HapticCoverMold (Autodesk Fusion 360 design; units mm, degrees)
Autodesk Fusion 360 part; units mm, degrees
sketch "Sketch1" plane through (0, 0, 0) normal (0, 0, 1) x (1, 0, 0) in component "Haptic Motor"
  circle A0 centre (0, 0) radius 5.2
  dimension "d1" = 10.4
  constraint coincident A0.centre origin
  measures "d1" diameter of A0
extrude "Extrude1" add sketch "Sketch1" along normal blind 6 makes body 1 in component "Haptic Motor"
sketch "Sketch1 (2)" plane through (0, 0, 0) normal (0, 0, 1) x (1, 0, 0) in component "Haptic Cover"
  circle A0 centre (0, 0) radius 5.2
  circle A1 centre (0, 0) radius 6.7
  dimension "d4" = 1.5
extrude "Extrude1'" add sketch "Sketch1 (2)" along normal blind 6 separate body makes body 2 in component "Haptic Cover"
extrude "Extrude2" add sketch "Sketch1 (2)" against normal blind 1.5 contours A0 | A1 bodies 2 in component "Haptic Cover"
sketch "Sketch1 (3)" plane through (0, 0, 0) normal (0, 1, 0) x (1, 0, 0) in component "Mold"
  line L0 (9.593, -10.0264) -> (-9.2463, -10.0264)
  line L1 (-9.2463, -10.0264) -> (-9.2463, 7.0138)
  line L2 (-9.2463, 7.0138) -> (9.593, 7.0138)
  line L3 (9.593, 7.0138) -> (9.593, -10.0264)
  constraint horizontal L0
  constraint vertical L1
  constraint horizontal L2
  constraint vertical L3
extrude "Extrude1''" add sketch "Sketch1 (3)" along normal mid plane 22 separate body makes body 3 in component "Mold"
ref_plane "WorkPlane1" through (0, 0, -1.5) normal (0, 0, -1) x (-1, 0, 0) in component "Mold"
combine "Combine1" operation cut target body 3 tool bodies 2 keep tools in component "Mold"
split "Split1" by plane through (0, 0, -1.5) normal (0, 0, -1) bodies 3 makes body 4 at (-2.9665, -3.6667, -7.0138) in component "Mold"
sketch "Sketch2" plane through (0, 0, -1.5) normal (0, 0, -1) x (1, 0, 0) in component "Mold"
  line L0 (9.593, 11) -> (-9.2463, 11)
  line L1 (-9.2463, 11) -> (-9.2463, -11)
  line L2 (-9.2463, -11) -> (9.593, -11)
  line L3 (9.593, -11) -> (9.593, 11)
  circle A0 centre (0, 0) radius 6.7
  line L4 (-3.9471, -7.9756) -> (-4.9947, -6.21)
  line L5 (-4.9947, -6.21) -> (-7.0475, -6.2343)
  line L6 (-7.0475, -6.2343) -> (-8.0529, -8.0244)
  line L7 (-8.0529, -8.0244) -> (-7.0053, -9.79)
  line L8 (-7.0053, -9.79) -> (-4.9525, -9.7657)
  line L9 (-4.9525, -9.7657) -> (-3.9471, -7.9756)
  line L10 (7.1755, 6.5257) -> (8.1675, 8.1105)
  line L11 (8.1675, 8.1105) -> (7.291, 9.7619)
  line L12 (7.291, 9.7619) -> (5.4226, 9.8287)
  line L13 (5.4226, 9.8287) -> (4.4306, 8.2439)
  line L14 (4.4306, 8.2439) -> (5.307, 6.5925)
  line L15 (5.307, 6.5925) -> (7.1755, 6.5257)
  line L16 (-8.3993, -8.0285) -> (-7.175, -10.0921)
  line L17 (-7.175, -10.0921) -> (-4.7757, -10.0636)
  line L18 (-4.7757, -10.0636) -> (-3.6007, -7.9715)
  line L19 (-3.6007, -7.9715) -> (-4.825, -5.9079)
  line L20 (-4.825, -5.9079) -> (-7.2243, -5.9364)
  line L21 (-7.2243, -5.9364) -> (-8.3993, -8.0285)
  line L22 (5.1232, 6.2988) -> (7.3378, 6.2197)
  line L23 (7.3378, 6.2197) -> (8.5136, 8.0981)
  line L24 (8.5136, 8.0981) -> (7.4748, 10.0555)
  line L25 (7.4748, 10.0555) -> (5.2602, 10.1346)
  line L26 (5.2602, 10.1346) -> (4.0844, 8.2563)
  line L27 (4.0844, 8.2563) -> (5.1232, 6.2988)
  point P0 (-6, -8)
  point P1 (6.299, 8.1772)
  dimension "d12" = 0.3
  dimension "d13" = 0.3
extrude "Extrude2'" add sketch "Sketch2" along normal blind 3 contours L4 L5 L6 L7 L8 L9 | L10 L11 L12 L13 L14 L15 bodies 3 in component "Mold"
extrude "Extrude3" cut sketch "Sketch2" along normal blind 3.3 contours L4 L5 L6 L7 L8 L9 | L10 L11 L12 L13 L14 L15 | L16 L17 L18 L19 L20 L21 | L22 L23 L24 L25 L26 L27 bodies 4 in component "Mold"
ref_plane "WorkPlane2" through (0.1734, 8, 4.2632) normal (0, 1, 0) x (0, 0, 1) in component "Mold"
component "Haptic Motor" placed x (1, 0, 0) y (0, 1, 0) z (0, 0, 1) at (0, 0, 0)
component "Haptic Cover" placed x (1, 0, 0) y (0, 1, 0) z (0, 0, 1) at (0, 0, 0)
component "Mold" placed x (1, 0, 0) y (0, 1, 0) z (0, 0, 1) at (0, 0, 0)
